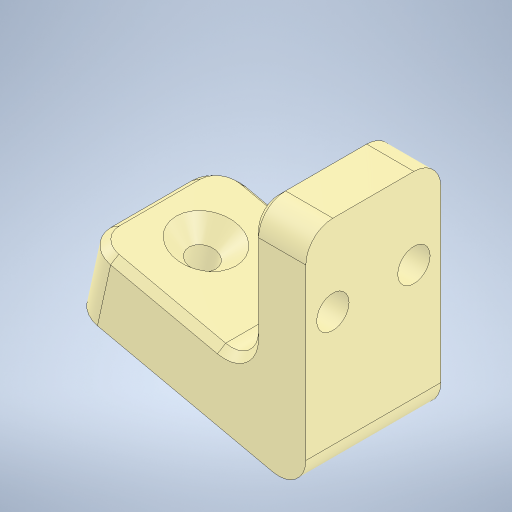
# Autodesk Inventor part: Spring Stand
Saved by Autodesk Inventor 2023.4 (Build 274418000, 418)
## iProperties
Created: 2024-05-07
Part Number: Spring Stand
Material: Nylon 6/6
Document SubType Name: Modeling
Designer: Nathan Cai
Density: 1.13 g/cm^3
Appearance: Nylon 6
Mass: 5.60032 g
Surface Area: 20.6997 cm^2
Volume: 4.95603 cm^3
Author: Nathan Cai
Autodesk Inventor part; units mm, degrees
ref_plane "YZ Plane" through (0, 0, 0) normal (1, 0, 0) x (0, 1, 0)
ref_plane "XZ Plane" through (0, 0, 0) normal (0, 1, 0) x (-1, 0, 0)
ref_plane "XY Plane" through (0, 0, 0) normal (0, 0, 1) x (1, 0, 0)
sketch "Sketch1" plane through (0, 0, 0) normal (0, 0, 1) x (1, 0, 0)
  line L0 (0, 0) -> (-28.575, 0)
  line L1 (-28.575, 0) -> (-28.575, -25.4) construction
  line L2 (-28.575, -25.4) -> (0, -25.4)
  line L3 (0, -25.4) -> (0, 0)
  line L4 (-28.575, -25.4) -> (-22.944, 0)
  line L5 (0, -25.4) -> (-27.2364, -19.3618)
  line L6 (-6.35, 0) -> (-6.35, -17.4881)
  line L7 (-6.35, -17.4881) -> (-25.862, -13.1624)
  dimension "d0" = 28.575
  dimension "d1" = 25.4
  dimension "d2" = 12.5
  dimension "d32" = 6.35
  dimension "d33" = 6.35
  constraints: 16 end point, 4 point on line, 3 parallel, 3 perpendicular, 1 horizontal
  measures "d0" distance of L2.end L1.end
  measures "d1" distance of L1.end L0.end
  measures "d2" angle of L1 L4
  measures "d32" distance between parallel lines of L5 L7
  measures "d33" distance between parallel lines of L3 L6
extrude "Extrusion1" add sketch "Sketch1" along normal blind 15.875 contours L3 L5 L4 L7 L6 L0
sketch "Sketch2" plane through (0, -25.4, 0) normal (-0.2164396, -0.976296, 0) x (0.976296, -0.2164396, 0)
  line L0 (-5.4976, 0) -> (-11.697, 0) projected
  line L1 (-21.5477, 0) -> (-21.5477, 15.875) construction
  line L2 (-5.4976, 15.875) -> (-11.697, 15.875) projected
  line L3 (-27.8977, 0) -> (-27.8977, 15.875) projected
  point P0 (-21.5477, 7.9375)
  dimension "d5" = 6.35
  constraints: 2 end point, 2 point on line, 1 midpoint, 1 vertical
  measures "d5" distance between parallel lines of L3 L1
hole "Hole1" at (-21.0369, -20.7362, 7.9375) direction (0.2164396, 0.976296, 0) diameter 3.2004 end through all clearance for "Socket Head Cap Screw" size "M3" standard "Ansi Metric M Profile"
thicken "Thicken1" operation add thickness 1.5875 both sides no extend neighbours yes toward (-0.2164396, -0.976296, 0) faces at (-6.4953, -23.96, 8.0018)
fillet "Fillet1" radius 3.175 2 edges at (0, -27.026, 7.9375) (-6.35, -17.4881, 7.9375)
sketch "Sketch4" plane through (0, 0, 15.875) normal (1, 0, 0) x (0, 0, -1)
  line L0 (15.875, -13.1624) -> (15.875, -20.9117) projected
  line L1 (15.875, -9.525) -> (0, -9.525) construction
  line L2 (0, -13.1624) -> (0, -20.9117) projected
  circle A0 centre (12.7, -9.525) radius 1.905
  line L3 (15.875, 0) -> (0, 0) projected
  circle A1 centre (3.175, -9.525) radius 1.905
  point P0 (15.875, -2.4878)
  point P1 (0, -2.4878)
  point P2 (7.9375, -9.525)
  dimension "d23" = 3.81
  dimension "d24" = 9.525
  dimension "d25" = 4.7625
  dimension "d28" = 360
  constraints: 3 point on line, 2 centre point, 2 end point, 1 horizontal, 1 midpoint, 5 other
  measures "d23" diameter of A0
  measures "d24" distance between parallel lines of L3 L1
  measures "d25" distance of point (7.937, -9.525) A0.centre
extrude "Extrusion2" cut sketch "Sketch4" against normal blind 9.525
fillet "Fillet2" radius 3.175 4 edges at (-26.721, -17.037, 0) (-26.721, -17.037, 15.875) (-3.175, 0, 0) (-3.175, 0, 15.875)
chamfer "Chamfer1" distance 0.7937 angle 45 12 edges at (-16.4872, -15.2407, 0) (-24.9541, -13.3636, 0.9299) (-25.862, -13.1624, 7.9375) (-24.9541, -13.3636, 14.9451) (-16.4872, -15.2407, 15.875) (-7.5377, -16.0082, 15.875) (-6.35, -8.3535, 15.875) (-6.35, -0.9299, 14.9451) (-6.35, 0, 7.9375) (-6.35, -0.9299, 0.9299) (-6.35, -8.3535, 0) (-7.5377, -16.0082, 0)
chamfer "Chamfer2" distance 2 angle 45 1 edges at (-19.6625, -14.5368, 9.5377)
body "Solid1"
